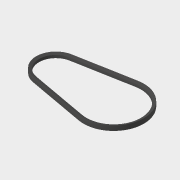
# Autodesk Inventor part: PWTR-0130
Saved by Autodesk Inventor 2021.1 (Build 251245000, 245)
## iProperties
Created: 2020-09-01
Part Number: PWTR-0130
Material: Rubber
Document SubType Name: Modeling
Designer: alid
Density: 0.93 g/cm^3
Appearance: Rubber - Black
Description: High Capacity Drive Belt
Author: alid
Revision Number: A
Autodesk Inventor part; units mm, degrees
ref_plane "YZ Plane" through (0, 0, 0) normal (1, 0, 0) x (0, 1, 0)
ref_plane "XZ Plane" through (0, 0, 0) normal (0, 1, 0) x (-1, 0, 0)
ref_plane "XY Plane" through (0, 0, 0) normal (0, 0, 1) x (1, 0, 0)
sketch "Sketch2" plane through (0, 0, 0) normal (0, 0, 1) x (1, 0, 0)
  line L0 (0, 62.5) -> (0, -62.5) construction
  arc A0 (-39.3467, 69.7) -> (39.3467, 69.7) centre (0, 62.5) ccw construction
  arc A1 (61.4792, -51.25) -> (-61.4792, -51.25) centre (0, -62.5) ccw construction
  line L1 (61.4792, -51.25) -> (39.3467, 69.7)
  line L2 (-61.4792, -51.25) -> (-39.3467, 69.7)
  arc A2 (39.3467, 69.7) -> (-39.3467, 69.7) centre (0, 62.5) ccw
  arc A3 (-61.4792, -51.25) -> (61.4792, -51.25) centre (0, -62.5) ccw
  line L3 (0, 62.5) -> (0, 102.5) construction
  point P0 (0, 0)
  point P1 (0, 0)
  dimension "d1" = 125
  dimension "d2" = 80
  dimension "d3" = 125
  constraints: 9 point on circle, 8 end point, 4 centre point, 4 tangent, 3 coincident, 1 midpoint, 1 vertical
  measures "d1" distance of L0.start L0.end
  measures "d2" diameter of A0
  measures "d3" diameter of A1
sketch "Sketch3" plane through (0, 0, 0) normal (1, 0, 0) x (0, 1, 0)
  line L0 (104.9986, 0) -> (98.9986, 0) construction
  line L1 (102.5, 4.25) -> (102.5, -4.25) construction
  line L2 (104.9986, 5.1594) -> (104.9986, -5.1594)
  line L3 (104.9986, -5.1594) -> (98.9986, -2.9756)
  line L4 (98.9986, -2.9756) -> (98.9986, 2.9756)
  line L5 (98.9986, 2.9756) -> (104.9986, 5.1594)
  point P0 (0, 0)
  point P1 (0, 0)
  point P2 (102.5, 0)
  point P3 (102.5, 0)
  point P4 (102.5, 0)
  dimension "d4" = 8.5
  dimension "d5" = 2.4986
  dimension "d6" = 40
  dimension "d7" = 6
  constraints: 12 end point, 3 midpoint, 2 coincident, 2 parallel, 2 point on line, 1 perpendicular, 1 vertical
  measures "d4" distance of L1.start L1.end
  measures "d5" distance between parallel lines of L2 L1
  measures "d6" angle of L5 L3
  measures "d7" distance between parallel lines of L4 L2
sweep "Sweep1" add profiles "Sketch3" path "Sketch2"
equation "\"d4\" = d8"
equation "\"d5\" = d9"
equation "\"d6\" = d10"
equation "\"d7\" = d11"
equation "\"d8\" = 8.5"
equation "\"d9\" = 2.49859"
equation "\"d10\" = 40deg"
equation "\"d11\" = 6"
body "Solid1"
